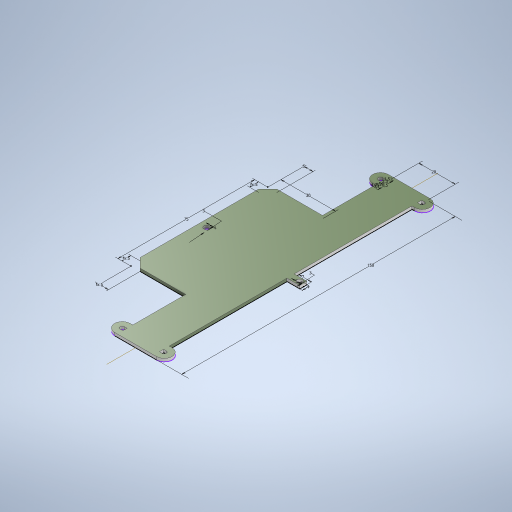
# Autodesk Inventor part: linefollower_chassy_model
Saved by Autodesk Inventor 2024 (Build 280153000, 153)
## iProperties
Created: 2024-02-06
Part Number: linefollower_chassy_model
Material: Generic
Document SubType Name: Modeling
Designer: kamil
Density: 1 g/cm^3
Appearance: Default
Author: kamil
Autodesk Inventor part; units mm, degrees
ref_plane "YZ Plane" through (0, 0, 0) normal (1, 0, 0) x (0, 1, 0)
ref_plane "XZ Plane" through (0, 0, 0) normal (0, 1, 0) x (-1, 0, 0)
ref_plane "XY Plane" through (0, 0, 0) normal (0, 0, 1) x (1, 0, 0)
sketch "Sketch1" plane through (0, 0, 0) normal (0, 1, 0) x (-1, 0, 0)
  line L0 (10, 75) -> (-10, 75)
  line L1 (-10, 75) -> (-10, -75)
  line L2 (-10, -75) -> (10, -75)
  line L3 (10, -75) -> (10, 75)
  line L4 (-10, 75) -> (10, -75) construction
  line L5 (-10, -75) -> (10, 75) construction
  line L6 (10, -75) -> (10, -67)
  line L7 (0, 75) -> (0, -75) construction
  line L8 (-10, 0) -> (10, 0) construction
  line L9 (10, -20.5447) -> (10, 19.5447)
  line L10 (10, 37.5) -> (35, 37.5)
  line L11 (40, 32.5) -> (40, -32.5)
  line L12 (35, -37.5) -> (10, -37.5)
  line L13 (10, -37.5) -> (10, 37.5)
  line L14 (-10, 2) -> (-17, 2)
  line L15 (-17, 2) -> (-17, -2)
  line L16 (-17, -2) -> (-10, -2)
  line L17 (-10, -2) -> (-10, 2)
  circle A0 centre (-15, 0) radius 1.5
  line L18 (35, -37.5) -> (40, -32.5)
  line L19 (35, 37.5) -> (40, 32.5)
  line L20 (10, -75) -> (11.51, -75)
  line L21 (10, -66.5) -> (11.51, -66.5)
  arc A1 (11.51, -75) -> (11.51, -66.5) centre (11.51, -70.75) ccw
  line L22 (10, -69.6) -> (11.5, -69.6)
  line L23 (10, -71.9) -> (11.5, -71.9)
  arc A2 (11.5, -71.9) -> (11.5, -69.6) centre (11.5, -70.75) ccw
  line L24 (-10, -75) -> (-11.51, -75)
  line L25 (-10, -66.5) -> (-11.51, -66.5)
  arc A3 (-11.51, -66.5) -> (-11.51, -75) centre (-11.51, -70.75) ccw
  line L26 (-10, -69.6) -> (-11.5, -69.6)
  line L27 (-10, -71.9) -> (-11.5, -71.9)
  arc A4 (-11.5, -69.6) -> (-11.5, -71.9) centre (-11.5, -70.75) ccw
  line L28 (10, 75) -> (11.51, 75)
  line L29 (10, 66.5) -> (11.51, 66.5)
  arc A5 (11.51, 66.5) -> (11.51, 75) centre (11.51, 70.75) ccw
  line L30 (10, 69.6) -> (11.5, 69.6)
  line L31 (10, 71.9) -> (11.5, 71.9)
  arc A6 (11.5, 69.6) -> (11.5, 71.9) centre (11.5, 70.75) ccw
  line L32 (-10, 71.9) -> (-11.5, 71.9)
  line L33 (-10, 69.6) -> (-11.5, 69.6)
  line L34 (-10, 66.5) -> (-11.51, 66.5)
  line L35 (-10, 75) -> (-11.51, 75)
  arc A7 (-11.5, 71.9) -> (-11.5, 69.6) centre (-11.5, 70.75) ccw
  arc A8 (-11.51, 75) -> (-11.51, 66.5) centre (-11.51, 70.75) ccw
  circle A9 centre (36, 0) radius 1.5
  point P0 (0, 0)
  point P1 (0, 0)
  point P2 (0, 0)
  point P3 (40, -37.5)
  point P4 (40, 37.5)
  point P5 (40, 0)
  point P6 (0, 0)
  point P7 (-13.5, -2)
  point P8 (-17, 0)
  point P9 (-10, 0)
  point P10 (10, -37.5)
  point P11 (10, -71)
  point P12 (10.755, -66.5)
  point P13 (10.75, -69.6)
  point P14 (-10.755, -66.5)
  point P15 (-10.75, -69.6)
  point P16 (10.755, 66.5)
  point P17 (10.75, 69.6)
  point P18 (-10.75, 69.6)
  point P19 (-10.755, 66.5)
  point P20 (10, -66.5)
  dimension "d1" = 20
  dimension "d5" = 30
  dimension "d6" = 75
  dimension "d7" = 3
  dimension "d8" = 4
  dimension "d9" = 7
  dimension "d10" = 5
  dimension "d11" = 5
  dimension "d12" = 5
  dimension "d13" = 5
  dimension "d14" = 5
  dimension "d18" = 1.51
  dimension "d19" = 8.5
  dimension "d22" = 4.25
  dimension "d23" = 1.5
  dimension "d24" = 3.1
  dimension "d25" = 2.3
  dimension "d26" = 150
  dimension "d27" = 3
  dimension "d28" = 4
  constraints: 72 end point, 33 symmetric about line, 16 point on circle, 14 midpoint, 11 point on line, 10 centre point, 6 horizontal, 6 parallel, 4 perpendicular, 3 horizontal alignment, 1 coincident, 6 other
  measures "d1" distance between parallel lines of L1 L3
  measures "d5" distance of point (40, -37.5) L12.end
  measures "d6" distance of point (40, 37.5) point (40, -37.5)
  measures "d7" diameter of A0
  measures "d8" distance from line of point (-13.5, -2) L14
  measures "d9" distance between parallel lines of L1 L15
  measures "d10" distance of point (-10, 0) A0.centre
  measures "d11" distance of L12.start point (40, -37.5)
  measures "d12" distance of L11.end point (40, -37.5)
  measures "d13" distance of L10.end point (40, 37.5)
  measures "d14" distance of L11.start point (40, 37.5)
  measures "d18" distance of L2.end L20.end
  measures "d19" distance between parallel lines of L20 L21
  measures "d22" distance from line of L21 A1.centre
  measures "d23" distance of L22.start L22.end
  measures "d24" distance of point (10.755, -66.5) point (10.75, -69.6)
  measures "d25" distance between parallel lines of L23 L22
  measures "d26" distance of L0.end L1.end
  measures "d27" diameter of A9
  measures "d28" distance from line of A9.centre L11
extrude "Extrusion1" add sketch "Sketch1" along normal blind 1.57 contours L3 L2 L1 L0 | L28 A5 L29 L3 L30 A6 L31 | L1 L32 A7 L33 L34 A8 L35 | L10 L19 L11 L18 L12 L3 | L1 L16 L15 L14 | L1 L26 A4 L27 L24 A3 L25 | L21 A1 L20 L3 L23 A2 L22
equation "\"d12\" = d11"
equation "\"d13\" = d11"
equation "\"d14\" = d13"
body "Solid1"
